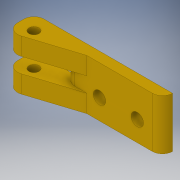
# Autodesk Inventor part: Upper_Spring_Hanger
Saved by Autodesk Inventor 2018.2 (Build 222227000, 227)
## iProperties
Created: 2018-03-24
Part Number: Upper_Spring_Hanger
Material: Generic
Document SubType Name: Modeling
Designer: MIABo
Density: 1 g/cm^3
Appearance: Default
Mass: 9.92112 g
Surface Area: 52.8908 cm^2
Volume: 9.92112 cm^3
Author: MIABo
## iProperties of the stored document Upper_Spring_Hanger_3DPrint.ipt
Created: 2018-03-27
Part Number: Upper_Spring_Hanger_3DPrint
Material: Generic
Document SubType Name: Modeling
Designer: MIABo
Density: 1 g/cm^3
Appearance: Default
Author: MIABo
Autodesk Inventor part; units mm, degrees
ref_plane "YZ Plane" through (0, 0, 0) normal (1, 0, 0) x (0, 1, 0)
ref_plane "XZ Plane" through (0, 0, 0) normal (0, 1, 0) x (-1, 0, 0)
ref_plane "XY Plane" through (0, 0, 0) normal (0, 0, 1) x (1, 0, 0)
sketch "Sketch1" plane through (0, 0, 0) normal (0, 0, 1) x (1, 0, 0)
  line L0 (-34.925, -12.7) -> (34.925, -12.7)
  line L1 (34.925, -12.7) -> (34.925, 12.7)
  line L2 (34.925, 12.7) -> (-34.925, 12.7)
  line L3 (-34.925, 12.7) -> (-34.925, -12.7)
  line L4 (-34.925, -12.7) -> (34.925, 12.7) construction
  line L5 (34.925, -12.7) -> (-34.925, 12.7) construction
  point P0 (0, 0)
  dimension "d0" = 25.4
  dimension "d1" = 69.85
  constraints: 12 end point, 2 midpoint, 2 parallel, 1 horizontal, 1 perpendicular
  measures "d0" distance of L2.end L0.start
  measures "d1" distance of L1.end L2.end
extrude "Extrusion1" add sketch "Sketch1" along normal blind 5.08
sketch "Sketch2" plane through (0, 0, 5.08) normal (0, 0, 1) x (1, 0, 0)
  line L0 (-34.925, 12.7) -> (-34.925, -12.7) projected
  line L1 (34.925, -12.7) -> (34.925, 12.7) projected
  line L2 (34.925, 12.7) -> (-34.925, 12.7) projected
  point P0 (0, 0)
  point P1 (3.175, -2.54)
  point P2 (22.225, -2.54)
  dimension "d5" = 12.7
  dimension "d6" = 15.24
  dimension "d7" = 15.24
  dimension "d18" = 19.05
  measures "d5" distance from line of L1 point (22.225, -2.54)
  measures "d6" distance from line of L2 point (22.225, -2.54)
  measures "d7" distance from line of L2 point (3.175, -2.54)
  measures "d18" distance of point (22.225, -2.54) point (3.175, -2.54)
hole "Hole1" at (3.175, -2.54, 5.08) at (22.225, -2.54, 5.08) direction (0, 0, -1) diameter 6.35 end through all
sketch "Sketch5" plane through (0, 0, 5.08) normal (0, 0, 1) x (1, 0, 0)
  line L0 (34.925, 12.7) -> (-34.925, 12.7) projected
  line L1 (-34.925, 12.7) -> (-14.2875, 12.7)
  line L2 (-14.2875, 12.7) -> (-14.2875, 3.81)
  line L3 (-14.2875, 3.81) -> (-34.925, 3.81)
  line L4 (-34.925, 3.81) -> (-34.925, 12.7)
  line L5 (-34.925, 12.7) -> (-34.925, -12.7) projected
  line L6 (-34.925, -12.7) -> (-14.2875, -12.7)
  line L7 (-14.2875, -12.7) -> (-14.2875, -3.81)
  line L8 (-14.2875, -3.81) -> (-34.925, -3.81)
  line L9 (-34.925, -3.81) -> (-34.925, -12.7)
  point P0 (0, 0)
  dimension "d19" = 7.62
  constraints: 16 end point, 4 parallel, 2 horizontal, 2 perpendicular, 1 collinear, 1 point on line
  measures "d19" distance between parallel lines of L8 L3
extrude "Extrusion2" add sketch "Sketch5" along normal blind 10.16
sketch "Sketch7" plane through (0, 0, 5.08) normal (0, 0, 1) x (1, 0, 0)
  line L0 (-29.845, 3.81) -> (-34.925, 3.81) projected
  line L1 (-19.3675, -3.81) -> (-14.2875, -3.81) projected
  line L2 (-34.925, 3.81) -> (-14.2875, 3.81)
  line L3 (-14.2875, 3.81) -> (-14.2875, -3.81)
  line L4 (-14.2875, -3.81) -> (-34.925, -3.81)
  line L5 (-34.925, -3.81) -> (-34.925, 3.81)
  point P0 (0, 0)
  constraints: 8 end point, 2 parallel, 1 horizontal, 1 perpendicular
extrude "Extrusion4" cut sketch "Sketch7" against normal blind 12.7
fillet "Fillet2" radius 5.08 2 edges at (-34.925, 8.255, 0) (-34.925, -8.255, 0)
sketch "Sketch8" plane through (34.925, -12.7, 0) normal (0, -1, 0) x (1, 0, 0)
  line L0 (-69.85, 5.08) -> (-69.85, 15.24) projected
  line L1 (-64.77, 0) -> (0, 0) projected
  point P0 (-34.925, 0)
  point P1 (-62.23, 7.62)
  point P2 (-69.85, 10.16)
  dimension "d28" = 7.62
  dimension "d29" = 7.62
  measures "d28" distance from line of point (-62.23, 7.62) L0
  measures "d29" distance from line of L1 point (-62.23, 7.62)
hole "Hole2" at (-27.305, -12.7, 7.62) direction (0, 1, 0) diameter 5.08 end through all
sketch "Sketch9" plane through (34.925, 12.7, 5.08) normal (0, 1, 0) x (1, 0, 0)
  line L0 (-49.2125, -10.16) -> (-69.85, -10.16) projected
  line L1 (-69.85, -10.16) -> (-38.1, 0)
  line L2 (-49.2125, 0) -> (0, 0) projected
  line L3 (-38.1, -10.16) -> (-38.1, 0)
  line L4 (-38.1, -10.16) -> (-69.85, -10.16)
  line L5 (-38.1, 0) -> (-58.7375, 0)
  line L6 (-58.7375, 0) -> (-58.7375, -6.604)
  point P0 (-34.925, 5.08)
  constraints: 10 end point, 3 point on line, 2 perpendicular, 1 vertical
extrude "Extrusion5" cut sketch "Sketch9" against normal through all contours L0 L1 L3 L4
extrude "Extrusion6" add sketch "Sketch9" against normal up to surface (8.89 mm away) contours L6 L5 L2 L1
fillet "Fillet3" radius 5.08 1 edges at (-34.925, 8.255, 15.24)
fillet "Fillet4" radius 5.08 1 edges at (-34.925, -8.255, 15.24)
extrude "Extrusion7" add sketch "Sketch9" along normal up to surface (8.89 mm away) from surface at -25.4 contours L6 L5 L2 L1
fillet "Fillet5" radius 5.08 1 edges at (34.925, 0, 5.08)
fillet "Fillet6" radius 5.08 1 edges at (-14.2875, 0, 5.08)
equation "\"d6\" = d7"
body "Solid1"
